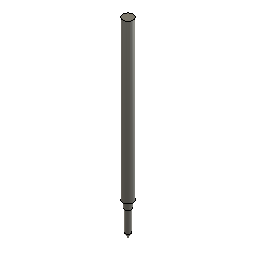
pen final v4 (Autodesk Fusion 360 archive; units mm, degrees)
design "Pen blank"
Autodesk Fusion 360 part; units mm, degrees
sketch "Sketch1" plane through (0, 0, 0) normal (0, 1, 0) x (1, 0, 0)
  circle A0 centre (0, 0) radius 3
  dimension "d1" = 6
  constraint coincident A0.centre origin
  measures "d1" diameter of A0
extrude "Extrude1" add sketch "Sketch1" along normal blind 91
sketch "Sketch2" plane through (0, 0, 0) normal (0, -1, 0) x (1, 0, 0)
  circle A0 centre (0, 0) radius 3
  circle A1 centre (0, 0) radius 2
  dimension "d4" = 4
  constraint coincident A0.centre A1.centre
  measures "d4" diameter of A1
extrude "Extrude2" add sketch "Sketch2" along normal blind 4 contours A1
sketch "Sketch3" plane through (0, -4, 0) normal (0, -1, 0) x (1, 0, 0)
  circle A0 centre (0, 0) radius 2
  circle A1 centre (0, 0) radius 1.5
  dimension "d7" = 3
  constraint concentric A0 A1
  measures "d7" diameter of A1
extrude "Extrude3" add sketch "Sketch3" along normal blind 17 contours A1
chamfer "Chamfer1" distance 0.5 angle 45 1 edges at (-1.3985, -4, 0.5424)
extrude "Extrude4" cut 1 faces at (0.567, -21, -0.5383) along direction (0, 1, 0) blind 1.5
chamfer "Chamfer3" distance 1.5 angle 65 1 edges at (-1.3985, -19.5, 0.5424) measured on face at (0.567, -19.5, -0.5383)
equation "d13 = 19.5 mm - 21.00 mm"
